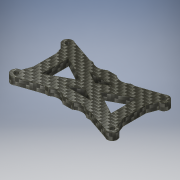
# Autodesk Inventor part: BottomBatteryBracket
Saved by Autodesk Inventor 2018 (Build 220112000, 112)
## iProperties
Created: 2018-08-26
Part Number: BottomBatteryBracket
Material: Generic
Document SubType Name: Modeling
Designer: anirudh
Density: 1 g/cm^3
Appearance: Carbon Fiber 1
Author: anirudh
Autodesk Inventor part; units mm, degrees
ref_plane "YZ Plane" through (0, 0, 0) normal (1, 0, 0) x (0, 1, 0)
ref_plane "XZ Plane" through (0, 0, 0) normal (0, 1, 0) x (-1, 0, 0)
ref_plane "XY Plane" through (0, 0, 0) normal (0, 0, 1) x (1, 0, 0)
sketch "Sketch1" plane through (0, 0, 0) normal (0, 1, 0) x (-1, 0, 0)
  line L0 (82.4144, -22.7348) -> (82.4144, -12.5748)
  line L1 (82.4144, -12.5748) -> (82.4144, -32.8948)
  line L2 (3.175, -12.7) -> (3.175, -33.02)
  circle A0 centre (85.2424, 0) radius 1.8
  circle A1 centre (85.2424, -45.72) radius 1.8
  circle A2 centre (0, 0) radius 1.8
  circle A3 centre (0, -45.72) radius 1.8
  arc A4 (85.2424, -4.445) -> (82.5491, 3.5361) centre (85.2424, 0) ccw
  arc A5 (82.5491, -49.2561) -> (85.2424, -41.275) centre (85.2424, -45.72) ccw
  arc A6 (2.6933, 3.5361) -> (0, -4.445) centre (0, 0) ccw
  arc A7 (0, -41.275) -> (2.6933, -49.2561) centre (0, -45.72) ccw
  line L3 (54.4604, -12.065) -> (30.782, -12.065)
  line L4 (54.4604, -33.655) -> (30.782, -33.655)
  line L5 (12.065, -12.7) -> (12.065, -33.02)
  line L6 (0, -4.445) -> (3.175, -12.7)
  line L7 (3.175, -33.02) -> (0, -41.275)
  line L8 (2.6933, 3.5361) -> (22.5806, -3.175)
  line L9 (2.6933, -49.2561) -> (22.5806, -42.545)
  line L10 (82.5491, -49.2561) -> (62.6618, -42.545)
  line L11 (82.4144, -32.8948) -> (85.2424, -41.275)
  line L12 (82.4144, -12.5748) -> (85.2424, -4.445)
  line L13 (73.5244, -12.5748) -> (73.5244, -32.8948)
  line L14 (82.5491, 3.5361) -> (62.6618, -3.175)
  line L15 (73.5244, -10.73) -> (50.9087, -22.86)
  line L16 (42.6212, -27.305) -> (30.782, -33.655)
  line L17 (30.782, -12.065) -> (42.6212, -18.415)
  line L18 (50.9087, -22.86) -> (73.5244, -34.99)
  line L19 (12.065, -10.9161) -> (34.3337, -22.86)
  line L20 (42.6212, -27.305) -> (54.4604, -33.655)
  line L21 (54.4604, -12.065) -> (42.6212, -18.415)
  line L22 (34.3337, -22.86) -> (12.065, -34.8039)
  line L23 (73.5244, -12.5748) -> (73.5244, -10.73)
  line L24 (73.5244, -32.8948) -> (73.5244, -34.99)
  line L25 (12.065, -12.7) -> (12.065, -10.9161)
  line L26 (12.065, -33.02) -> (12.065, -34.8039)
  arc A8 (46.9121, -3.175) -> (59.6409, -3.175) centre (53.2765, 3.9116) ccw
  arc A9 (25.9485, -3.175) -> (38.6773, -3.175) centre (32.3129, 3.9116) ccw
  line L27 (62.6618, -3.175) -> (59.6409, -3.175)
  line L28 (46.9121, -3.175) -> (38.6773, -3.175)
  line L29 (25.9485, -3.175) -> (22.5806, -3.175)
  arc A10 (59.6409, -42.545) -> (46.9121, -42.545) centre (53.2765, -49.6316) ccw
  arc A11 (38.6773, -42.545) -> (25.9485, -42.545) centre (32.3129, -49.6316) ccw
  line L30 (62.6618, -42.545) -> (59.6409, -42.545)
  line L31 (46.9121, -42.545) -> (38.6773, -42.545)
  line L32 (25.9485, -42.545) -> (22.5806, -42.545)
  constraints: 66 end point, 16 point on circle, 12 centre point, 9 parallel, 6 horizontal, 4 coincident, 3 vertical, 2 point on line, 1 perpendicular
extrude "Extrusion3" add sketch "Sketch1" along normal blind 6.35
body "Solid3"
